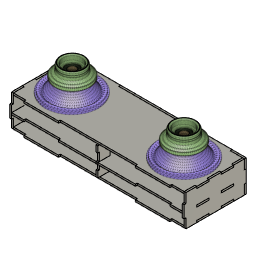
Groove Coaster v14 (Autodesk Fusion 360 design; units mm, degrees)
Autodesk Fusion 360 part; units mm, degrees
sketch "box_top-6mm" plane through (0, 0, 0) normal (0, 0, 1) x (1, 0, 0)
  line L0 (1457.4056, 711.1292) -> (1344.9056, 711.1292)
  line L1 (936.4056, 550.1292) -> (942.4056, 550.1292)
  line L2 (1094.9056, 705.1292) -> (1094.9056, 711.1292)
  line L3 (1503.4056, 670.1292) -> (1497.4056, 670.1292)
  line L4 (1344.9056, 711.1292) -> (1344.9056, 705.1292)
  line L5 (1344.9056, 509.1292) -> (1457.4056, 509.1292)
  line L6 (942.4056, 515.1292) -> (982.4056, 515.1292)
  line L7 (1503.4056, 590.1292) -> (1497.4056, 590.1292)
  line L8 (1503.4056, 630.1292) -> (1503.4056, 670.1292)
  line L9 (936.4056, 670.1292) -> (936.4056, 630.1292)
  line L10 (982.4056, 509.1292) -> (1094.9056, 509.1292)
  line L11 (1457.4056, 705.1292) -> (1457.4056, 711.1292)
  line L12 (1094.9056, 509.1292) -> (1094.9056, 515.1292)
  line L13 (982.4056, 705.1292) -> (942.4056, 705.1292)
  line L14 (942.4056, 705.1292) -> (942.4056, 670.1292)
  circle A0 centre (1037.4056, 610.1292) radius 82.5
  line L15 (1457.4056, 509.1292) -> (1457.4056, 515.1292)
  line L16 (1503.4056, 550.1292) -> (1503.4056, 590.1292)
  line L17 (982.4056, 711.1292) -> (982.4056, 705.1292)
  line L18 (936.4056, 630.1292) -> (942.4056, 630.1292)
  line L19 (1497.4056, 630.1292) -> (1503.4056, 630.1292)
  line L20 (1497.4056, 550.1292) -> (1503.4056, 550.1292)
  line L21 (942.4056, 630.1292) -> (942.4056, 590.1292)
  line L22 (1497.4056, 670.1292) -> (1497.4056, 705.1292)
  line L23 (942.4056, 670.1292) -> (936.4056, 670.1292)
  line L24 (1497.4056, 590.1292) -> (1497.4056, 630.1292)
  line L25 (1094.9056, 711.1292) -> (982.4056, 711.1292)
  line L26 (1344.9056, 705.1292) -> (1094.9056, 705.1292)
  line L27 (1094.9056, 515.1292) -> (1344.9056, 515.1292)
  circle A1 centre (1402.4056, 610.1292) radius 82.5
  line L28 (1497.4056, 705.1292) -> (1457.4056, 705.1292)
  line L29 (1497.4056, 515.1292) -> (1497.4056, 550.1292)
  line L30 (1344.9056, 515.1292) -> (1344.9056, 509.1292)
  line L31 (936.4056, 590.1292) -> (936.4056, 550.1292)
  line L32 (942.4056, 590.1292) -> (936.4056, 590.1292)
  line L33 (1457.4056, 515.1292) -> (1497.4056, 515.1292)
  line L34 (982.4056, 515.1292) -> (982.4056, 509.1292)
  line L35 (942.4056, 550.1292) -> (942.4056, 515.1292)
extrude "Extrude2" add sketch "box_top-6mm" along normal blind 6 makes body 1
move_body "Move1" bodies 1 to x (1, 0, 0) y (0, 1, 0) z (0, 0, 1) at (0, 0, 125)
sketch "box_middle-6mm" plane through (0, 0, 0) normal (0, 0, 1) x (1, 0, 0)
  circle A0 centre (1015.4056, 569.1292) radius 1.5
  line L0 (942.4056, 670.1292) -> (936.4056, 670.1292)
  line L1 (1344.9056, 705.1292) -> (1344.9056, 711.1292)
  line L2 (942.4056, 711.1292) -> (942.4056, 670.1292)
  line L3 (1503.4056, 550.1292) -> (1503.4056, 590.1292)
  line L4 (1457.4056, 515.1292) -> (1457.4056, 509.1292)
  line L5 (1094.9056, 515.1292) -> (1094.9056, 509.1292)
  circle A1 centre (1380.4056, 569.1292) radius 1.5
  line L6 (936.4056, 670.1292) -> (936.4056, 630.1292)
  circle A2 centre (1037.4056, 610.1292) radius 20
  circle A3 centre (1402.4056, 610.1292) radius 20
  line L7 (942.4056, 509.1292) -> (982.4056, 509.1292)
  line L8 (1497.4056, 509.1292) -> (1497.4056, 550.1292)
  line L9 (1094.9056, 705.1292) -> (982.4056, 705.1292)
  circle A4 centre (1424.4056, 569.1292) radius 1.5
  circle A5 centre (1059.4056, 569.1292) radius 1.5
  line L10 (942.4056, 590.1292) -> (936.4056, 590.1292)
  line L11 (936.4056, 630.1292) -> (942.4056, 630.1292)
  line L12 (936.4056, 590.1292) -> (936.4056, 550.1292)
  circle A6 centre (1015.4056, 651.1292) radius 1.5
  line L13 (1497.4056, 670.1292) -> (1497.4056, 711.1292)
  line L14 (1344.9056, 515.1292) -> (1457.4056, 515.1292)
  line L15 (1503.4056, 630.1292) -> (1503.4056, 670.1292)
  circle A7 centre (1059.4056, 651.1292) radius 1.5
  line L16 (1503.4056, 590.1292) -> (1497.4056, 590.1292)
  circle A8 centre (1424.4056, 651.1292) radius 1.5
  line L17 (1216.9056, 711.1292) -> (1094.9056, 711.1292)
  line L18 (936.4056, 550.1292) -> (942.4056, 550.1292)
  line L19 (942.4056, 630.1292) -> (942.4056, 590.1292)
  circle A9 centre (1380.4056, 651.1292) radius 1.5
  line L20 (982.4056, 711.1292) -> (942.4056, 711.1292)
  line L21 (982.4056, 509.1292) -> (982.4056, 515.1292)
  line L22 (1457.4056, 509.1292) -> (1497.4056, 509.1292)
  line L23 (1503.4056, 670.1292) -> (1497.4056, 670.1292)
  line L24 (1094.9056, 509.1292) -> (1216.9056, 509.1292)
  line L25 (1344.9056, 509.1292) -> (1344.9056, 515.1292)
  line L26 (1457.4056, 711.1292) -> (1457.4056, 705.1292)
  line L27 (982.4056, 705.1292) -> (982.4056, 711.1292)
  line L28 (982.4056, 515.1292) -> (1094.9056, 515.1292)
  line L29 (1222.9056, 711.1292) -> (1222.9056, 690.1292)
  line L30 (1094.9056, 711.1292) -> (1094.9056, 705.1292)
  line L31 (1216.9056, 509.1292) -> (1216.9056, 530.1292)
  line L32 (1222.9056, 509.1292) -> (1344.9056, 509.1292)
  line L33 (1497.4056, 590.1292) -> (1497.4056, 630.1292)
  line L34 (1216.9056, 690.1292) -> (1216.9056, 711.1292)
  line L35 (1497.4056, 711.1292) -> (1457.4056, 711.1292)
  line L36 (1216.9056, 530.1292) -> (1222.9056, 530.1292)
  line L37 (1497.4056, 550.1292) -> (1503.4056, 550.1292)
  line L38 (1222.9056, 530.1292) -> (1222.9056, 509.1292)
  line L39 (1344.9056, 711.1292) -> (1222.9056, 711.1292)
  line L40 (1457.4056, 705.1292) -> (1344.9056, 705.1292)
  line L41 (942.4056, 550.1292) -> (942.4056, 509.1292)
  line L42 (1222.9056, 690.1292) -> (1216.9056, 690.1292)
  line L43 (1497.4056, 630.1292) -> (1503.4056, 630.1292)
extrude "Extrude3" add sketch "box_middle-6mm" along normal blind 6 separate body makes body 2
move_body "Move2" bodies 2 to x (1, 0, 0) y (0, 1, 0) z (0, 0, 1) at (0, 0, 30)
move_body "Move3" bodies 1 to x (1, 0, 0) y (0, 1, 0) z (0, 0, 1) at (0, 0, -60)
sketch "box_front-6mm" plane through (0, 0, 0) normal (0, 1, 0) x (1, 0, 0)
  line L0 (1497.4056, 589.9528) -> (1497.4056, 611.4528)
  line L1 (1222.9056, 654.9528) -> (1216.9056, 654.9528)
  line L2 (982.4056, 558.9528) -> (982.4056, 564.9528)
  line L3 (1457.4056, 564.9528) -> (1457.4056, 558.9528)
  line L4 (1503.4056, 589.9528) -> (1497.4056, 589.9528)
  line L5 (1457.4056, 617.4528) -> (1497.4056, 617.4528)
  line L6 (936.4056, 558.9528) -> (982.4056, 558.9528)
  line L7 (1222.9056, 634.9528) -> (1222.9056, 654.9528)
  line L8 (1503.4056, 558.9528) -> (1503.4056, 589.9528)
  line L9 (1497.4056, 611.4528) -> (1457.4056, 611.4528)
  line L10 (1216.9056, 634.9528) -> (1222.9056, 634.9528)
  line L11 (1216.9056, 654.9528) -> (1216.9056, 634.9528)
  line L12 (982.4056, 564.9528) -> (1094.9056, 564.9528)
  line L13 (1457.4056, 558.9528) -> (1503.4056, 558.9528)
  line L14 (1457.4056, 611.4528) -> (1457.4056, 617.4528)
  line L15 (936.4056, 589.9528) -> (936.4056, 558.9528)
  line L16 (1497.4056, 617.4528) -> (1497.4056, 629.9528)
  line L17 (1344.9056, 558.9528) -> (1344.9056, 564.9528)
  line L18 (1094.9056, 564.9528) -> (1094.9056, 558.9528)
  line L19 (1094.9056, 558.9528) -> (1344.9056, 558.9528)
  line L20 (982.4056, 617.4528) -> (982.4056, 611.4528)
  line L21 (1344.9056, 654.9528) -> (1344.9056, 660.9528)
  line L22 (1503.4056, 660.9528) -> (1457.4056, 660.9528)
  line L23 (1094.9056, 611.4528) -> (1344.9056, 611.4528)
  line L24 (942.4056, 589.9528) -> (936.4056, 589.9528)
  line L25 (1457.4056, 654.9528) -> (1344.9056, 654.9528)
  line L26 (1094.9056, 660.9528) -> (1094.9056, 654.9528)
  line L27 (1094.9056, 617.4528) -> (1094.9056, 611.4528)
  line L28 (936.4056, 660.9528) -> (936.4056, 629.9528)
  line L29 (942.4056, 629.9528) -> (942.4056, 617.4528)
  line L30 (1344.9056, 564.9528) -> (1457.4056, 564.9528)
  line L31 (942.4056, 617.4528) -> (982.4056, 617.4528)
  line L32 (1216.9056, 564.9528) -> (1222.9056, 564.9528)
  line L33 (982.4056, 660.9528) -> (936.4056, 660.9528)
  line L34 (1094.9056, 654.9528) -> (982.4056, 654.9528)
  line L35 (1497.4056, 629.9528) -> (1503.4056, 629.9528)
  line L36 (1344.9056, 611.4528) -> (1344.9056, 617.4528)
  line L37 (1457.4056, 660.9528) -> (1457.4056, 654.9528)
  line L38 (942.4056, 611.4528) -> (942.4056, 589.9528)
  line L39 (936.4056, 629.9528) -> (942.4056, 629.9528)
  line L40 (1222.9056, 584.9528) -> (1216.9056, 584.9528)
  line L41 (1222.9056, 564.9528) -> (1222.9056, 584.9528)
  line L42 (1344.9056, 617.4528) -> (1094.9056, 617.4528)
  line L43 (1216.9056, 584.9528) -> (1216.9056, 564.9528)
  line L44 (982.4056, 611.4528) -> (942.4056, 611.4528)
  line L45 (982.4056, 654.9528) -> (982.4056, 660.9528)
  line L46 (1344.9056, 660.9528) -> (1094.9056, 660.9528)
  line L47 (1503.4056, 629.9528) -> (1503.4056, 660.9528)
extrude "Extrude4" add sketch "box_front-6mm" along normal blind 6 separate body makes body 3
move_body "Move4" bodies 3 to x (1, 0, 0) y (0, 1, 0) z (0, 0, 1) at (0, 560, 600)
move_body "Move5" bodies 3 to x (1, 0, 0) y (0, 1, 0) z (0, 0, 1) at (0, -50, 60)
move_body "Move6" bodies 3 to x (1, 0, 0) y (0, 1, 0) z (0, 0, 1) at (0, -0.89, 0.9559)
move_body "Move7" bodies 2 to x (1, 0, 0) y (0, 1, 0) z (0, 0, 1) at (0, 0, 13.5)
move_body "Move8" bodies 1 to x (1, 0, 0) y (0, 1, 0) z (0, 0, 1) at (0, 0, 30)
move_body "Move9" bodies 1 to x (1, 0, 0) y (0, 1, 0) z (0, 0, 1) at (0, 0, 1)
sketch "box_bottom-6mm" plane through (0, 0, 0) normal (0, 0, 1) x (1, 0, 0)
  line L0 (1503.4056, 550.1292) -> (1503.4056, 590.1292)
  line L1 (1503.4056, 590.1292) -> (1497.4056, 590.1292)
  line L2 (1497.4056, 630.1292) -> (1503.4056, 630.1292)
  line L3 (1503.4056, 630.1292) -> (1503.4056, 670.1292)
  line L4 (1503.4056, 670.1292) -> (1497.4056, 670.1292)
  line L5 (1344.9056, 515.1292) -> (1344.9056, 509.1292)
  line L6 (942.4056, 705.1292) -> (942.4056, 670.1292)
  line L7 (942.4056, 590.1292) -> (936.4056, 590.1292)
  line L8 (942.4056, 515.1292) -> (982.4056, 515.1292)
  line L9 (936.4056, 670.1292) -> (936.4056, 630.1292)
  line L10 (1457.4056, 509.1292) -> (1457.4056, 515.1292)
  line L11 (1497.4056, 590.1292) -> (1497.4056, 630.1292)
  line L12 (1094.9056, 711.1292) -> (982.4056, 711.1292)
  line L13 (936.4056, 590.1292) -> (936.4056, 550.1292)
  line L14 (1344.9056, 711.1292) -> (1344.9056, 705.1292)
  line L15 (1497.4056, 515.1292) -> (1497.4056, 550.1292)
  line L16 (982.4056, 705.1292) -> (942.4056, 705.1292)
  line L17 (1344.9056, 705.1292) -> (1094.9056, 705.1292)
  line L18 (982.4056, 509.1292) -> (1094.9056, 509.1292)
  line L19 (1094.9056, 509.1292) -> (1094.9056, 515.1292)
  line L20 (982.4056, 515.1292) -> (982.4056, 509.1292)
  line L21 (1497.4056, 550.1292) -> (1503.4056, 550.1292)
  line L22 (942.4056, 670.1292) -> (936.4056, 670.1292)
  line L23 (1497.4056, 705.1292) -> (1457.4056, 705.1292)
  line L24 (1457.4056, 515.1292) -> (1497.4056, 515.1292)
  line L25 (942.4056, 630.1292) -> (942.4056, 590.1292)
  line L26 (1094.9056, 515.1292) -> (1344.9056, 515.1292)
  line L27 (1344.9056, 509.1292) -> (1457.4056, 509.1292)
  line L28 (936.4056, 630.1292) -> (942.4056, 630.1292)
  line L29 (942.4056, 550.1292) -> (942.4056, 515.1292)
  line L30 (1457.4056, 711.1292) -> (1344.9056, 711.1292)
  line L31 (1457.4056, 705.1292) -> (1457.4056, 711.1292)
  line L32 (1497.4056, 670.1292) -> (1497.4056, 705.1292)
  line L33 (936.4056, 550.1292) -> (942.4056, 550.1292)
  line L34 (982.4056, 711.1292) -> (982.4056, 705.1292)
  line L35 (1094.9056, 705.1292) -> (1094.9056, 711.1292)
extrude "Extrude6" add sketch "box_bottom-6mm" along normal blind 6 separate body makes body 4
sketch "box_front-USBC-6mm" plane through (0, 0, 0) normal (0, 0, 1) x (1, 0, 0)
  line L0 (1503.4056, 558.9528) -> (1503.4056, 589.9528)
  line L1 (1222.9056, 654.9528) -> (1216.9056, 654.9528)
  line L2 (1216.9056, 634.9528) -> (1222.9056, 634.9528)
  line L3 (1457.4056, 654.9528) -> (1344.9056, 654.9528)
  line L4 (1457.4056, 611.4528) -> (1457.4056, 617.4528)
  line L5 (1216.9056, 654.9528) -> (1216.9056, 634.9528)
  line L6 (1094.9056, 558.9528) -> (1344.9056, 558.9528)
  line L7 (1457.4056, 617.4528) -> (1497.4056, 617.4528)
  line L8 (1497.4056, 629.9528) -> (1503.4056, 629.9528)
  line L9 (1344.9056, 564.9528) -> (1457.4056, 564.9528)
  line L10 (1497.4056, 589.9528) -> (1497.4056, 611.4528)
  line L11 (982.4056, 660.9528) -> (936.4056, 660.9528)
  line L12 (982.4056, 558.9528) -> (982.4056, 564.9528)
  line L13 (1094.9056, 564.9528) -> (1094.9056, 558.9528)
  line L14 (982.4056, 654.9528) -> (982.4056, 660.9528)
  line L15 (1094.9056, 617.4528) -> (1094.9056, 611.4528)
  line L16 (982.4056, 617.4528) -> (982.4056, 611.4528)
  line L17 (936.4056, 589.9528) -> (936.4056, 558.9528)
  line L18 (1457.4056, 660.9528) -> (1457.4056, 654.9528)
  line L19 (1344.9056, 654.9528) -> (1344.9056, 660.9528)
  line L20 (1503.4056, 629.9528) -> (1503.4056, 660.9528)
  line L21 (1503.4056, 660.9528) -> (1457.4056, 660.9528)
  line L22 (1497.4056, 611.4528) -> (1457.4056, 611.4528)
  line L23 (936.4056, 558.9528) -> (982.4056, 558.9528)
  line L24 (1497.4056, 617.4528) -> (1497.4056, 629.9528)
  line L25 (1503.4056, 589.9528) -> (1497.4056, 589.9528)
  line L26 (1344.9056, 558.9528) -> (1344.9056, 564.9528)
  line L27 (982.4056, 564.9528) -> (1094.9056, 564.9528)
  line L28 (1457.4056, 558.9528) -> (1503.4056, 558.9528)
  line L29 (1457.4056, 564.9528) -> (1457.4056, 558.9528)
  line L30 (1222.9056, 634.9528) -> (1222.9056, 654.9528)
  line L31 (936.4056, 660.9528) -> (936.4056, 629.9528)
  line L32 (1344.9056, 660.9528) -> (1094.9056, 660.9528)
  line L33 (942.4056, 589.9528) -> (936.4056, 589.9528)
  line L34 (982.4056, 611.4528) -> (942.4056, 611.4528)
  line L35 (942.4056, 617.4528) -> (982.4056, 617.4528)
  line L36 (1225.0756, 624.4228) -> (1214.7356, 624.4228)
  line L37 (942.4056, 611.4528) -> (942.4056, 589.9528)
  line L38 (1094.9056, 660.9528) -> (1094.9056, 654.9528)
  line L39 (1225.0756, 627.9828) -> (1225.0756, 624.4228)
  line L40 (936.4056, 629.9528) -> (942.4056, 629.9528)
  line L41 (1344.9056, 611.4528) -> (1344.9056, 617.4528)
  line L42 (1214.7356, 624.4228) -> (1214.7356, 627.9828)
  line L43 (942.4056, 629.9528) -> (942.4056, 617.4528)
  line L44 (1344.9056, 617.4528) -> (1094.9056, 617.4528)
  line L45 (1094.9056, 611.4528) -> (1344.9056, 611.4528)
  line L46 (1222.9056, 564.9528) -> (1222.9056, 584.9528)
  line L47 (1222.9056, 584.9528) -> (1216.9056, 584.9528)
  line L48 (1216.9056, 564.9528) -> (1222.9056, 564.9528)
  line L49 (1214.7356, 627.9828) -> (1225.0756, 627.9828)
  line L50 (1216.9056, 584.9528) -> (1216.9056, 564.9528)
  line L51 (1094.9056, 654.9528) -> (982.4056, 654.9528)
extrude "Extrude7" add sketch "box_front-USBC-6mm" along normal blind 6 separate body makes body 5
move_body "Move16" bodies 5 to x (1, 0, 0) y (0, 1, 0) z (0, 0, 1) at (0, 50, 0)
move_body "Move17" bodies 5 to x (1, 0, 0) y (0, 0, -1) z (0, 1, 0) at (0, 608.9528, 608.9528)
move_body "Move18" bodies 5 to x (1, 0, 0) y (0, 1, 0) z (0, 0, 1) at (0, 100, 100)
move_body "Align2" bodies 5 to x (1, 0, 0) y (0, 1, 0) z (0, 0, 1) at (0, -3.8236, 2)
sketch "box_side" plane through (0, 0, 0) normal (0, 0, 1) x (1, 0, 0)
  line L0 (37.7555, 99.9923) -> (2.7555, 99.9923)
  line L1 (77.7555, 94.9923) -> (37.7555, 94.9923)
  line L2 (192.7555, 99.9923) -> (157.7555, 99.9923)
  line L3 (117.7555, 94.9923) -> (117.7555, 99.9923)
  line L4 (2.7555, 99.9923) -> (2.7555, 69.9923)
  line L5 (2.7555, 69.9923) -> (-2.2445, 69.9923)
  line L6 (117.7555, 47.9923) -> (117.7555, 42.9923)
  line L7 (197.7555, 69.9923) -> (192.7555, 69.9923)
  line L8 (2.7555, -0.0077) -> (37.7555, -0.0077)
  line L9 (37.7555, 42.9923) -> (77.7555, 42.9923)
  line L10 (37.7555, 4.9923) -> (77.7555, 4.9923)
  line L11 (157.7555, 4.9923) -> (157.7555, -0.0077)
  line L12 (77.7555, 42.9923) -> (77.7555, 47.9923)
  line L13 (192.7555, 69.9923) -> (192.7555, 99.9923)
  line L14 (117.7555, 99.9923) -> (77.7555, 99.9923)
  line L15 (192.7555, 29.9923) -> (197.7555, 29.9923)
  line L16 (37.7555, 94.9923) -> (37.7555, 99.9923)
  line L17 (-2.2445, 29.9923) -> (2.7555, 29.9923)
  line L18 (117.7555, 42.9923) -> (157.7555, 42.9923)
  line L19 (157.7555, -0.0077) -> (192.7555, -0.0077)
  line L20 (117.7555, 4.9923) -> (157.7555, 4.9923)
  line L21 (157.7555, 99.9923) -> (157.7555, 94.9923)
  line L22 (2.7555, 29.9923) -> (2.7555, -0.0077)
  line L23 (197.7555, 29.9923) -> (197.7555, 69.9923)
  line L24 (157.7555, 47.9923) -> (117.7555, 47.9923)
  line L25 (-2.2445, 69.9923) -> (-2.2445, 29.9923)
  line L26 (77.7555, 4.9923) -> (77.7555, -0.0077)
  line L27 (37.7555, 47.9923) -> (37.7555, 42.9923)
  line L28 (157.7555, 94.9923) -> (117.7555, 94.9923)
  line L29 (77.7555, 47.9923) -> (37.7555, 47.9923)
  line L30 (117.7555, -0.0077) -> (117.7555, 4.9923)
  line L31 (37.7555, -0.0077) -> (37.7555, 4.9923)
  line L32 (77.7555, -0.0077) -> (117.7555, -0.0077)
  line L33 (192.7555, -0.0077) -> (192.7555, 29.9923)
  line L34 (157.7555, 42.9923) -> (157.7555, 47.9923)
  line L35 (77.7555, 99.9923) -> (77.7555, 94.9923)
extrude "Extrude8" add sketch "box_side" along normal blind 6 separate body contours L0 L1 L2 L3 L4 L5 L7 L8 L10 L11 L13 L14 L15 L16 L17 L19 L20 L21 L22 L23 L25 L26 L28 L30 L31 L32 L33 L35 | L6 L18 L24 L34 | L9 L12 L27 L29 makes body 6
move_body "Move19" bodies 5 1 2 4 3 to x (1, 0, 0) y (0, 1, 0) z (0, 0, 1) at (-1100, 0, 0)
move_body "Move20" bodies 1 2 4 3 5 to x (1, 0, 0) y (0, 1, 0) z (0, 0, 1) at (0, -800, 0)
move_body "Move21" bodies 6 to x (0, -1, 0) y (0, 0, 1) z (-1, 0, 0) at (-157.2445, -92.2522, 0.0077)
move_body "Move22" bodies 6 to x (1, 0, 0) y (0, 1, 0) z (0, 0, 1) at (0, 0, 10)
move_body "Align3" bodies 6 to x (1, 0, 0) y (0, 0, -1) z (0, 1, 0) at (-0.3499, -184.8708, -164.0077)
move_body "Move23" bodies 6 to x (1, 0, 0) y (0, 0, 1) z (0, -1, 0) at (0, -163.8708, 175.8708)
move_face "OffsetFaces1" offset 1 3 faces at (-159.5944, -106.5375, 1) (-159.5944, -183.2042, 1) (-161.5944, -261.5375, 1) on bodies 6
move_face "OffsetFaces2" offset 1 3 faces at (-161.5944, -118.2042, 101) (-161.5944, -196.5375, 101) (-161.5944, -273.2042, 101) on bodies 6
move_face "MoveFace1" by (0, 1, 0) 1 faces at (-159.5944, -89.8708, 57.6667) on bodies 6
move_face "MoveFace2" by (0, -1, 0) 1 faces at (-161.5944, -289.8708, 57.6667) on bodies 6
copy_body "CopyPasteBodies2" bodies 6 makes body 7
move_body "Move25" bodies 7 to x (1, 0, 0) y (0, 1, 0) z (0, 0, 1) at (561, 0, 0)
sketch "box_insert" plane through (0, 0, 0) normal (0, 0, 1) x (1, 0, 0)
  line L0 (5.1496, 37.1882) -> (10.1496, 37.1882)
  line L1 (10.1496, 37.1882) -> (10.1496, 19.1882)
  line L2 (45.1496, 37.1882) -> (25.1496, 37.1882)
  line L3 (10.1496, 42.1882) -> (5.1496, 42.1882)
  line L4 (45.1496, 89.1882) -> (5.1496, 89.1882)
  line L5 (5.1496, 19.1882) -> (5.1496, -0.8118)
  line L6 (5.1496, 42.1882) -> (5.1496, 37.1882)
  line L7 (25.1496, 42.1882) -> (45.1496, 42.1882)
  line L8 (25.1496, 37.1882) -> (25.1496, 42.1882)
  line L9 (10.1496, 69.1882) -> (10.1496, 42.1882)
  line L10 (5.1496, -0.8118) -> (45.1496, -0.8118)
  line L11 (45.1496, -0.8118) -> (45.1496, 37.1882)
  line L12 (5.1496, 69.1882) -> (10.1496, 69.1882)
  line L13 (5.1496, 89.1882) -> (5.1496, 69.1882)
  line L14 (10.1496, 19.1882) -> (5.1496, 19.1882)
  line L15 (45.1496, 42.1882) -> (45.1496, 89.1882)
extrude "Extrude9" add sketch "box_insert" along normal blind 6 separate body makes body 8
move_body "Move26" bodies 8 to x (0, -1, 0) y (0, 0, 1) z (-1, 0, 0) at (5.1496, -83.6622, 0.8118)
move_body "Move27" bodies 8 to x (1, 0, 0) y (0, 1, 0) z (0, 0, 1) at (120, 0, 5)
move_face "MoveFace3" by (0, 0, 1) 1 faces at (123.1496, -92.1451, 48) on bodies 8
move_body "Align4" bodies 8 to x (1, 0, 0) y (0, 1, 0) z (0, 0, 1) at (-2.2441, -0.059, 0.5)
move_face "MoveFace4" by (0, 0, 0.5) 1 faces at (118.9056, -115.5375, 5.5) on bodies 8
move_face "MoveFace5" by (0, 0, 0.5) 1 faces at (120.9056, -92.2042, 25.5) on bodies 8
move_face "MoveFace6" by (0, 0, 0.5) 1 faces at (120.9056, -115.5375, 95.5) on bodies 8
move_face "MoveFace7" by (0, 0, 0.5) 1 faces at (120.9056, -90.5375, 75.5) on bodies 8
move_face "MoveFace8" by (0, 0, -0.5) 1 faces at (118.9056, -122.2042, 43.5) on bodies 8
move_face "MoveFace9" by (0, 0, 0.5) 1 faces at (120.9056, -115.5375, 48.5) on bodies 8
move_face "MoveFace10" by (0, 0, 0.5) 1 faces at (120.9056, -115.5375, 49) on bodies 8
move_face "MoveFace11" by (0, 0, 0.5) 1 faces at (118.9056, -122.2042, 43) on bodies 8
copy_body "CopyPasteBodies3" bodies 8 makes body 9
move_body "Move30" bodies 9 to x (-1, 0, 0) y (0, -1, 0) z (0, 0, 1) at (233.8111, -377.7417, 0)
move_body "Move31" bodies 9 to x (1, 0, 0) y (0, 1, 0) z (0, 0, 1) at (5, 0, 0)
move_body "Align6" bodies 9 to x (1, 0, 0) y (0, 1, 0) z (0, 0, 1) at (1, -2, 0)
move_face "MoveFace13" by (0, -4, 0) 1 faces at (120.9056, -93.8708, 37.6667) on bodies 8
move_face "MoveFace14" by (0, -1, 0) 1 faces at (120.9056, -97.8708, 37.6667) on bodies 8
other "Base Mesh Feature1"
other "Modify1"
other "Modify2"
other "Modify3"
other "Modify4"
other "Modify5"
other "Modify6"
other "Modify7"
other "CopyPasteMeshes1"
other "Modify8"
other "Base Mesh Feature3"
other "Base Mesh Feature4"
other "Modify9"
other "Modify10"
other "Modify11"
other "Modify12"
other "Modify13"
other "Modify14"
other "Modify15"
other "Modify16"
other "Modify17"
other "Modify18"
other "CopyPasteMeshes2"
other "Modify19"
other "Modify20"
other "Modify21"
other "Base Mesh Feature5"
other "Modify22"
other "Modify23"
other "Modify24"
other "Modify25"
other "Modify26"
other "Modify27"
other "Modify28"
other "Modify29"
other "CopyPasteMeshes3"
other "Modify30"
other "Modify31"
other "Modify32"
other "Modify33"
hidden bodies 3
named bodies: "Top", "Center_Horz", "Front", "bottom", "back+usbc", "left", "right", "backinsert", "frontinsert"
